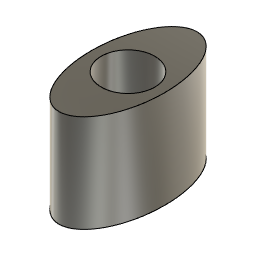
7.3 Intersect sketch (Autodesk Fusion 360 design; units mm, degrees)
Autodesk Fusion 360 part; units mm, degrees
sketch "Sketch1" plane through (0, 0, 0) normal (0, 0, 1) x (1, 0, 0)
  ellipse E0 centre (0, 0) end of major axis (0, 31.5965) minor radius 16.6986
  line L0 (0, -31.5965) -> (0, 31.5965)
  line L1 (16.6986, 0) -> (-16.6986, 0)
  constraint coincident E0.centre origin
  constraint vertical L0
  constraint coincident E0 L0.start
  constraint coincident E0 L0.end
  constraint coincident E0 L1.start
  constraint coincident E0 L1.end
extrude "Extrude1" add sketch "Sketch1" along normal blind 44.585
ref_plane "WorkPlane1" through (0, 0, 13.758) normal (0, 0, 1) x (1, 0, 0)
sketch "Sketch9" plane through (0, 0, 44.585) normal (0, 0, 1) x (-1, 0, 0)
  circle A0 centre (0, 0) radius 12.2459
  constraint coincident A0.centre origin
extrude "Extrude3" cut sketch "Sketch9" against normal blind 43.276
